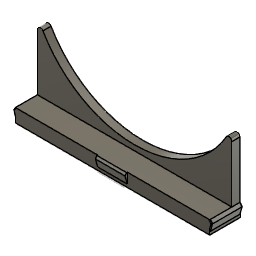
Wemos D1 mini pro Box closure (Autodesk Fusion 360 design; units mm, degrees)
Autodesk Fusion 360 part; units mm, degrees
note: some values were not read from the file. Set by a fixed rule: which sketch regions a step uses.
sketch "Esquisse1" plane through (0, 0, 0) normal (0, 1, 0) x (1, 0, 0)
  line L0 (-13.2, 2.1) -> (13.2, 2.1)
  line L1 (13.2, 2.1) -> (13.2, -2.1)
  line L2 (13.2, -2.1) -> (-13.2, -2.1)
  line L3 (-13.2, -2.1) -> (-13.2, 2.1)
  line L4 (-13.2, -2.1) -> (13.2, 2.1) construction
  dimension "d1" = 26.4
  dimension "d2" = 4.2
  constraint horizontal L0
  constraint vertical L1
  constraint horizontal L2
  constraint vertical L3
  constraint midpoint origin L4
  measures "d1" distance of L0.start L0.end
  measures "d2" distance of L0.start L2.end
extrude "Extrusion1" add sketch "Esquisse1" along normal blind 1.4 draft 16
sketch "Esquisse2" plane through (0, 0, 0) normal (0, -1, 0) x (1, 0, 0)
  line L0 (13.2, 2.1) -> (-13.2, 2.1)
  line L1 (-13.2, 2.1) -> (-13.2, -2.1)
  line L2 (-13.2, -2.1) -> (13.2, -2.1)
  line L3 (13.2, -2.1) -> (13.2, 2.1)
  line L4 (-2.0144, 2.1) -> (-15, 2.1)
  line L5 (-15, 2.1) -> (-15, 3.5)
  line L6 (-15, 3.5) -> (-2.0144, 3.5)
  line L7 (-2.0144, 3.5) -> (-2.0144, 2.1)
  line L8 (0, 0) -> (-16.5, 0) construction
  line L9 (0, 0) -> (0, 9) construction
  line L10 (-15, -3.5) -> (-2.0144, -3.5)
  line L11 (-15, -2.1) -> (-15, -3.5)
  line L12 (-2.0144, -2.1) -> (-15, -2.1)
  line L13 (-2.0144, -3.5) -> (-2.0144, -2.1)
  line L14 (2.0144, 3.5) -> (2.0144, 2.1)
  line L15 (15, 3.5) -> (2.0144, 3.5)
  line L16 (15, 2.1) -> (15, 3.5)
  line L17 (2.0144, 2.1) -> (15, 2.1)
  line L18 (2.0144, -2.1) -> (15, -2.1)
  line L19 (15, -3.5) -> (2.0144, -3.5)
  line L20 (2.0144, -3.5) -> (2.0144, -2.1)
  line L21 (15, -2.1) -> (15, -3.5)
  point P0 (13.2, 2.1)
  point P1 (13.2, -2.1)
  constraint horizontal L4
  constraint vertical L5
  constraint horizontal L6
  constraint vertical L7
  constraint coincident L0 L4.start
  constraint coincident L8.start L9.start
  constraint horizontal L8
  constraint perpendicular L8 L9
  constraint symmetric L4.start L8 L12.start
  constraint symmetric L4.end L8 L11.start
  constraint symmetric L5.end L8 L10.start
  constraint symmetric L6.end L8 L10.end
  constraint symmetric L0.end L9 P0
  constraint symmetric L1.end L9 P1
  constraint symmetric L4.start L9 L14.end
  constraint symmetric L4.end L9 L16.start
  constraint symmetric L5.end L9 L15.start
  constraint symmetric L6.end L9 L14.start
  constraint symmetric L9 L10.start L19.start
  constraint symmetric L9 L10.end L19.end
  constraint symmetric L9 L11.start L18.end
  constraint symmetric L9 L12.start L18.start
extrude "Extrusion2" cut sketch "Esquisse2" against normal blind 2.5 contours L0 L14 L15 L16 L17 | L2 L18 L19 L20 L21 | L0 L4 L5 L6 L7 | L2 L10 L11 L12 L13
sketch "Esquisse3" plane through (0, 1.4, 0) normal (0, 1, 0) x (-1, 0, 0)
  line L0 (-2.0144, 2.5014) -> (-2.0144, 2.1)
  line L1 (-2.0144, 2.1) -> (-13.6014, 2.1)
  line L2 (-13.6014, 2.1) -> (-13.6014, -2.1)
  line L3 (-13.6014, -2.1) -> (-2.0144, -2.1)
  line L4 (-2.0144, -2.1) -> (-2.0144, -2.5014)
  line L5 (-2.0144, -2.5014) -> (2.0144, -2.5014)
  line L6 (2.0144, -2.5014) -> (2.0144, -2.1)
  line L7 (2.0144, -2.1) -> (13.6014, -2.1)
  line L8 (13.6014, -2.1) -> (13.6014, 2.1)
  line L9 (13.6014, 2.1) -> (2.0144, 2.1)
  line L10 (2.0144, 2.1) -> (2.0144, 2.5014)
  line L11 (2.0144, 2.5014) -> (-2.0144, 2.5014)
  line L12 (13.2, -0.9) -> (-13.2, -0.9)
  line L13 (-13.2, -0.9) -> (-13.2, -2)
  line L14 (-13.2, -2) -> (13.2, -2)
  line L15 (13.2, -2) -> (13.2, -0.9)
  line L16 (0, 0) -> (0, -0.9)
  dimension "d7" = 26.4
  dimension "d8" = 0.1
  dimension "d9" = 1.1
  constraint horizontal L12
  constraint vertical L13
  constraint horizontal L14
  constraint vertical L15
  constraint coincident L16.start origin
  constraint midpoint L12 L16.end
  constraint vertical L16
  measures "d7" distance of L13.end L14.end
  measures "d8" distance of L3 L14
  measures "d9" distance of L12 L14
extrude "Extrusion3" add sketch "Esquisse3" along normal blind 9 contours L12 L13 L14 L15
sketch "Esquisse4" plane through (0, 0, -0.9) normal (0, 0, 1) x (1, 0, 0)
  line L0 (-13.2, 1.4) -> (13.2, 1.4)
  line L1 (13.2, 1.4) -> (13.2, 10.4)
  line L2 (13.2, 10.4) -> (-13.2, 10.4)
  line L3 (-13.2, 10.4) -> (-13.2, 1.4)
  circle A0 centre (0, 16.5) radius 14.389
  line L4 (0, 16.5) -> (0, 0) construction
  constraint coincident A0.centre L4.start
  constraint coincident L4.end origin
  constraint perpendicular L0 L4
extrude "Extrusion4" cut sketch "Esquisse4" against normal blind 6 contours L2 A0 picked at (2.5741, 8.3863)
sketch "Esquisse5" plane through (0, 0, -2) normal (0, 0, -1) x (-1, 0, 0)
  line L0 (-13.2, 10.4) -> (-13.2, 1.4)
  line L1 (-13.2, 1.4) -> (13.2, 1.4)
  line L2 (13.2, 1.4) -> (13.2, 10.4)
  line L3 (-13.032, 10.4) -> (-13.2, 10.4)
  arc A0 (-13.032, 10.4) -> (13.032, 10.4) centre (0, 16.5) ccw
  circle A1 centre (-7.1, 6.9) radius 1.5
  line L4 (13.2, 10.4) -> (13.032, 10.4)
  point P0 (-13.2, 1.4)
  dimension "d16" = 3
  dimension "d17" = 6.1
  dimension "d18" = 5.5
  measures "d16" diameter of A1
  measures "d17" horizontal distance of A1.centre P0
  measures "d18" distance of L1 A1.centre
extrude "Extrusion5" add 1 faces at (-5.743, 0, 0.7) along direction (0, -1, 0) blind 0.4
chamfer "Chanfrein3" distance 0.4 angle 45 2 edges at (13.6014, 1.4, 0) (-13.6014, 1.4, 0)
chamfer "Chanfrein4" distance 0.3 angle 45 2 edges at (0, 1.4, -2.5014) (0, 1.4, 2.5014)
fillet "Congé1" radius 0.4 4 edges at (-13.2, 10.4, -1.45) (13.2, 10.4, -1.45) (13.032, 10.4, -1.45) (-13.032, 10.4, -1.45)
chamfer "Chanfrein5" distance 0.1 angle 45 8 edges at (-13.3456, 0.5077, 2.1) (-13.3463, 1.2077, 2.1) (-13.3456, 0.5077, -2.1) (-13.3463, 1.2077, -2.1) (13.3463, 1.2077, 2.1) (13.3456, 0.5077, 2.1) (13.3463, 1.2077, -2.1) (13.3456, 0.5077, -2.1)
